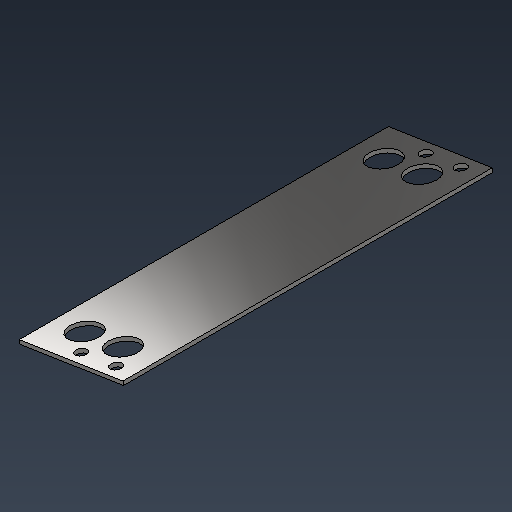
# Autodesk Inventor part: SteelFront
Saved by Autodesk Inventor 2026.2 (Build 302298010, 298A)
## iProperties
Created: 2026-04-07
Part Number: SteelFront
Material: Steel, Alloy
Document SubType Name: Modeling
Designer: szymo
Density: 7.73 g/cm^3
Appearance: Semi-Polished(2)
Mass: 19.4408 g
Surface Area: 54.2307 cm^2
Volume: 2.51498 cm^3
Author: szymo
Autodesk Inventor part; units mm, degrees
ref_plane "YZ Plane" through (0, 0, 0) normal (1, 0, 0) x (0, 1, 0)
ref_plane "XZ Plane" through (0, 0, 0) normal (0, 1, 0) x (-1, 0, 0)
ref_plane "XY Plane" through (0, 0, 0) normal (0, 0, 1) x (1, 0, 0)
sketch "Sketch1" plane through (0, 0, 0) normal (0, 0, 1) x (1, 0, 0)
  line L0 (0, -95.0088) -> (0, -82.1408) construction
  line L1 (2, -82.1408) -> (2, -91.0088) construction
  line L2 (2, -91.0088) -> (4, -91.0088) construction
  line L3 (4, -91.0088) -> (0, -95.0088) construction
  circle A0 centre (15.35, -55.1458) radius 14.7 construction
  line L4 (2.3528, -90.8088) -> (30.45, -86.4652)
  line L5 (30.45, -86.4652) -> (30.2972, -85.4769)
  line L6 (30.2972, -85.4769) -> (2.2, -89.8205)
  line L7 (2.2, -89.8205) -> (2.3528, -90.8088)
  line L8 (30.45, -86.4652) -> (30.45, -70.1877) construction
  line L9 (25, -86.2958) -> (4.5, -86.2958) projected
  line L10 (4.5, -86.2958) -> (4.5, -69.7958) projected
  line L11 (25, -69.7958) -> (4.5, -69.7958) projected
  line L12 (25, -86.2958) -> (25, -69.7958) projected
  line L13 (0, -82.1408) -> (2, -82.1408) projected
  dimension "d0" = 1
  dimension "d1" = 0.2
  dimension "d2" = 0.2
  dimension "d3" = 0.4
  dimension "d4" = 0
  constraints: 10 end point, 2 parallel, 1 perpendicular, 1 vertical
  measures "d0" distance between parallel lines of L6 L4
  measures "d1" distance from line of L1 L6.end
  measures "d2" distance from line of L2 L4.start
  measures "d3" distance edge to line of A0 L8
  measures "d4" distance from line of L6 L9.start
extrude "Extrusion1" add sketch "Sketch1" along normal mid plane 100 contours L7 L6 L5 L4
sketch "Sketch2" plane through (30.45, -86.4652, -50) normal (0.1527759, -0.9882609, 0) x (0.9882609, 0.1527759, 0)
  line L0 (-26.6096, 16.5) -> (-26.6096, 83.5) projected
  line L1 (-28.6334, 0) -> (-28.6334, 1) projected
  circle A0 centre (-5.2783, 96.6469) radius 1.5
  circle A1 centre (-14.8697, 96.6469) radius 1.5
  circle A2 centre (-14.8697, 3.3531) radius 1.5
  circle A3 centre (-5.2783, 3.3531) radius 1.5
  circle A4 centre (-9.5918, 90.5) radius 4
  circle A5 centre (-20.1476, 90.5) radius 4
  circle A6 centre (-9.5918, 9.5) radius 4
  circle A7 centre (-20.1476, 9.5) radius 4
  line L2 (-28.6334, 99) -> (-27.9959, 99) projected
  line L3 (-27.9959, 99) -> (-27.9959, 82.5) projected
  line L4 (-27.9959, 82.5) -> (-28.6334, 82.5) projected
  line L5 (-28.6334, 17.5) -> (-28.6334, 82.5) projected
  line L6 (-28.6334, 17.5) -> (-27.9959, 17.5) projected
  line L7 (-27.9959, 17.5) -> (-27.9959, 1) projected
  line L8 (-27.9959, 1) -> (-28.6334, 1) projected
  line L9 (-2.2739, 0) -> (-28.6334, 0) projected
  line L10 (-2.2739, 100) -> (-28.6334, 100) projected
  line L11 (-28.6334, 99) -> (-28.6334, 100) projected
  line L12 (-2.2739, 15.5) -> (-25.5977, 15.5) projected
  ellipse E0 centre (-25.5977, 16.5) end of major axis (-26.6096, 16.5) minor radius 1 (-26.6096, 16.5) -> (-25.5977, 15.5) ccw projected
  ellipse E1 centre (-25.5977, 83.5) end of major axis (-26.6096, 83.5) minor radius 1 (-25.5977, 84.5) -> (-26.6096, 83.5) ccw projected
  line L13 (-2.2739, 84.5) -> (-25.5977, 84.5) projected
  line L14 (-2.2739, 15.5) -> (-2.2739, 0) projected
  line L15 (-2.2739, 84.5) -> (-2.2739, 100) projected
  circle A8 centre (-5.2739, 95.7039) radius 2.25 projected
  circle A9 centre (-15.9797, 95.7039) radius 2.25 projected
  ellipse E2 centre (-21.2618, 90.5) end of major axis (-16.73, 90.5) minor radius 4.5 (-17.3352, 92.7467) -> (-17.3352, 88.2533) ccw projected
  line L16 (-17.3352, 92.7467) -> (-14.6243, 92.7467) projected
  ellipse E3 centre (-10.6977, 90.5) end of major axis (-6.1659, 90.5) minor radius 4.5 (-14.6243, 88.2533) -> (-14.6243, 92.7467) ccw projected
  line L17 (-14.6243, 88.2533) -> (-17.3352, 88.2533) projected
  circle A10 centre (-15.9797, 4.2961) radius 2.25 projected
  circle A11 centre (-5.2739, 4.2961) radius 2.25 projected
  ellipse E4 centre (-21.2618, 9.5) end of major axis (-16.73, 9.5) minor radius 4.5 (-17.3352, 11.7467) -> (-17.3352, 7.2533) ccw projected
  line L18 (-17.3352, 11.7467) -> (-14.6243, 11.7467) projected
  ellipse E5 centre (-10.6977, 9.5) end of major axis (-6.1659, 9.5) minor radius 4.5 (-14.6243, 7.2533) -> (-14.6243, 11.7467) ccw projected
  line L19 (-14.6243, 7.2533) -> (-17.3352, 7.2533) projected
  point P0 (-16.8827, 50)
  point P1 (-16.268, 88.2533)
  point P2 (-16.268, 92.7467)
  point P3 (-16.268, 7.2533)
  point P4 (-16.268, 11.7467)
  point P5 (-16.3079, 88.2533)
  point P6 (-16.3079, 92.7467)
  point P7 (-16.3079, 7.2533)
  point P8 (-16.3079, 11.7467)
  point P9 (-16.3688, 88.2533)
  point P10 (-16.3688, 92.7467)
  point P11 (-16.3688, 7.2533)
  point P12 (-16.3688, 11.7467)
  point P13 (-16.5217, 88.2533)
  point P14 (-16.5217, 92.7467)
  point P15 (-16.5217, 7.2533)
  point P16 (-16.5217, 11.7467)
  point P17 (-16.5463, 88.2533)
  point P18 (-16.5463, 92.7467)
  point P19 (-16.5463, 7.2533)
  point P20 (-16.5463, 11.7467)
  point P21 (-17.2602, 88.2533)
  point P22 (-17.2602, 92.7467)
  point P23 (-17.2602, 7.2533)
  point P24 (-17.2602, 11.7467)
  point P25 (-17.265, 88.2533)
  point P26 (-17.265, 92.7467)
  point P27 (-17.265, 7.2533)
  point P28 (-17.265, 11.7467)
  point P29 (-17.2698, 88.2533)
  point P30 (-17.2698, 92.7467)
  point P31 (-17.2698, 7.2533)
  point P32 (-17.2698, 11.7467)
  point P33 (-17.2746, 88.2533)
  point P34 (-17.2746, 92.7467)
  point P35 (-17.2746, 7.2533)
  point P36 (-17.2746, 11.7467)
  point P37 (-17.2794, 88.2533)
  point P38 (-17.2794, 92.7467)
  point P39 (-17.2794, 7.2533)
  point P40 (-17.2794, 11.7467)
  dimension "d7" = 3
  dimension "d8" = 3
  dimension "d9" = 3
  dimension "d10" = 3
  dimension "d13" = 8
  dimension "d14" = 8
  dimension "d15" = 8
  dimension "d16" = 8
  constraints: 8 centre point, 10 other
  measures "d7" diameter of A0
  measures "d8" diameter of A1
  measures "d9" diameter of A2
  measures "d10" diameter of A3
  measures "d13" diameter of A4
  measures "d14" diameter of A5
  measures "d15" diameter of A7
  measures "d16" diameter of A6
extrude "Extrusion2" cut sketch "Sketch2" against normal through all contours A0 A8 | A8 A0 | A1 A9 | A9 A1 | A2 A10 | A10 A2 | A3 A11 | A11 A3 | A4 E3 | E3 A4 | L16 E2 A5 | A5 L17 E2 L16 | A5 E2 L17 | A6 E5 | E5 A6 | L18 E4 A7 | A7 L19 E4 L18 | A7 E4 L19 picked at (-5.2254, 97.0136) picked at (-5.226, 98.0072) picked at (-13.9287, 97.077) picked at (-14.6647, 96.4433) picked at (-13.9287, 2.923) picked at (-14.6647, 3.5567) picked at (-5.2254, 2.9864) picked at (-5.226, 1.9928)
equation "\"d14\" = d13"
equation "\"d15\" = d13"
equation "\"d16\" = d13"
body "Solid1"
